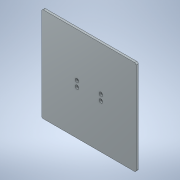
# Autodesk Inventor part: plate
Saved by Autodesk Inventor 2020 (Build 240168000, 168)
## iProperties
Created: 2026-07-10
Part Number: plate
Material: Iron, Cast
Document SubType Name: Modeling
Designer: drago
Density: 7.15 g/cm^3
Appearance: Zinc
Author: drago
Autodesk Inventor part; units mm, degrees
ref_plane "YZ Plane" through (0, 0, 0) normal (1, 0, 0) x (0, 1, 0)
ref_plane "XZ Plane" through (0, 0, 0) normal (0, 1, 0) x (-1, 0, 0)
ref_plane "XY Plane" through (0, 0, 0) normal (0, 0, 1) x (1, 0, 0)
sketch "Sketch1" plane through (0, 0, 0) normal (0, 0, 1) x (1, 0, 0)
  line L0 (-63, 65) -> (63, 65)
  line L1 (65, 63) -> (65, -63)
  line L2 (63, -65) -> (-63, -65)
  line L3 (-65, -63) -> (-65, 63)
  circle A0 centre (16.5, 4) radius 1
  circle A1 centre (-16.5, 4) radius 1
  circle A2 centre (-16.5, -4) radius 1
  circle A3 centre (16.5, -4) radius 1
  arc A4 (-63, 65) -> (-65, 63) centre (-63, 63) ccw
  arc A5 (65, 63) -> (63, 65) centre (63, 63) ccw
  arc A6 (63, -65) -> (65, -63) centre (63, -63) ccw
  arc A7 (-65, -63) -> (-63, -65) centre (-63, -63) ccw
  dimension "d7" = 2
  constraints: 8 centre point, 8 end point, 8 point on circle, 8 tangent, 3 equal radius, 2 parallel, 1 horizontal, 1 perpendicular
  measures "d7" radius of A4
extrude "Extrusion1" add sketch "Sketch1" along normal blind 3
chamfer "Chamfer1" distance 1.5 angle 45 4 edges at (-17.5, 4, 3) (-17.5, -4, 3) (15.5, 4, 3) (15.5, -4, 3)
body "Solid1"
